DriveGear v1 (Autodesk Fusion 360 design; units mm, degrees)
Autodesk Fusion 360 part; units mm, degrees
note: some values were not read from the file. Set by a fixed rule: which sketch regions a step uses.
sketch "Sketch1" plane through (0, 0, 0) normal (0, 1, 0) x (1, 0, 0)
  line L0 (25.6646, 0) -> (28.2938, 0.0001)
  line L1 (28.2938, 0.0001) -> (28.3201, 0.001)
  line L2 (28.3201, 0.001) -> (28.3702, 0.0041)
  line L3 (28.3702, 0.0041) -> (28.4441, 0.0108)
  line L4 (28.4441, 0.0108) -> (28.5416, 0.0225)
  line L5 (28.5416, 0.0225) -> (28.6623, 0.0406)
  line L6 (28.6623, 0.0406) -> (28.806, 0.0665)
  line L7 (28.806, 0.0665) -> (28.9724, 0.1014)
  line L8 (28.9724, 0.1014) -> (29.1609, 0.1467)
  line L9 (29.1609, 0.1467) -> (29.3711, 0.2038)
  line L10 (29.3711, 0.2038) -> (29.6025, 0.2738)
  line L11 (29.6025, 0.2738) -> (29.8544, 0.3582)
  line L12 (29.8544, 0.3582) -> (30.1263, 0.4581)
  line L13 (30.1263, 0.4581) -> (30.4173, 0.5748)
  line L14 (30.4173, 0.5748) -> (30.7268, 0.7094)
  line L15 (30.7268, 0.7094) -> (31.0539, 0.8632)
  line L16 (31.0539, 0.8632) -> (31.3978, 1.0372)
  line L17 (31.3978, 1.0372) -> (31.7575, 1.2325)
  line L18 (31.7575, 1.2325) -> (32.132, 1.4503)
  line L19 (32.132, 1.4503) -> (32.5204, 1.6915)
  line L20 (32.5204, 1.6915) -> (32.9216, 1.9571)
  line L21 (32.9216, 1.9571) -> (33.3344, 2.248)
  line L22 (33.3344, 2.248) -> (33.7578, 2.5652)
  line L23 (33.7578, 2.5652) -> (34.1905, 2.9094)
  line L24 (34.1905, 2.9094) -> (34.6313, 3.2816)
  line L25 (34.6313, 3.2816) -> (35.0789, 3.6823)
  line L26 (35.0789, 3.6823) -> (35.532, 4.1124)
  line L27 (35.532, 4.1124) -> (35.9893, 4.5725)
  line L28 (35.9893, 4.5725) -> (36.4494, 5.0631)
  line L29 (36.4494, 5.0631) -> (36.6248, 5.5415)
  line L30 (36.6248, 5.5415) -> (36.4585, 6.5468)
  line L31 (36.4585, 6.5468) -> (36.1385, 6.9433)
  line L32 (36.1385, 6.9433) -> (35.5449, 7.2596)
  line L33 (35.5449, 7.2596) -> (34.9638, 7.5479)
  line L34 (34.9638, 7.5479) -> (34.3963, 7.8092)
  line L35 (34.3963, 7.8092) -> (33.8435, 8.0445)
  line L36 (33.8435, 8.0445) -> (33.3063, 8.2548)
  line L37 (33.3063, 8.2548) -> (32.7858, 8.4414)
  line L38 (32.7858, 8.4414) -> (32.2829, 8.6054)
  line L39 (32.2829, 8.6054) -> (31.7983, 8.7479)
  line L40 (31.7983, 8.7479) -> (31.333, 8.8702)
  line L41 (31.333, 8.8702) -> (30.8876, 8.9734)
  line L42 (30.8876, 8.9734) -> (30.4629, 9.059)
  line L43 (30.4629, 9.059) -> (30.0595, 9.1282)
  line L44 (30.0595, 9.1282) -> (29.6779, 9.1822)
  line L45 (29.6779, 9.1822) -> (29.3187, 9.2224)
  line L46 (29.3187, 9.2224) -> (28.9824, 9.2502)
  line L47 (28.9824, 9.2502) -> (28.6692, 9.267)
  line L48 (28.6692, 9.267) -> (28.3797, 9.274)
  line L49 (28.3797, 9.274) -> (28.114, 9.2727)
  line L50 (28.114, 9.2727) -> (27.8724, 9.2646)
  line L51 (27.8724, 9.2646) -> (27.655, 9.2509)
  line L52 (27.655, 9.2509) -> (27.4619, 9.2331)
  line L53 (27.4619, 9.2331) -> (27.2932, 9.2126)
  line L54 (27.2932, 9.2126) -> (27.1488, 9.1908)
  line L55 (27.1488, 9.1908) -> (27.0287, 9.169)
  line L56 (27.0287, 9.169) -> (26.9327, 9.1488)
  line L57 (26.9327, 9.1488) -> (26.8606, 9.1314)
  line L58 (26.8606, 9.1314) -> (26.8121, 9.1182)
  line L59 (26.8121, 9.1182) -> (26.7868, 9.1106)
  line L60 (26.7868, 9.1106) -> (24.2977, 8.264)
  line L61 (24.2977, 8.264) -> (22.2262, 12.8323)
  line L62 (22.2262, 12.8323) -> (24.5031, 14.1469)
  line L63 (24.5031, 14.1469) -> (24.5254, 14.1609)
  line L64 (24.5254, 14.1609) -> (24.5673, 14.1887)
  line L65 (24.5673, 14.1887) -> (24.6279, 14.2314)
  line L66 (24.6279, 14.2314) -> (24.7064, 14.2903)
  line L67 (24.7064, 14.2903) -> (24.802, 14.3664)
  line L68 (24.802, 14.3664) -> (24.9135, 14.4606)
  line L69 (24.9135, 14.4606) -> (25.0401, 14.574)
  line L70 (25.0401, 14.574) -> (25.1807, 14.7075)
  line L71 (25.1807, 14.7075) -> (25.3342, 14.862)
  line L72 (25.3342, 14.862) -> (25.4996, 15.0384)
  line L73 (25.4996, 15.0384) -> (25.6756, 15.2374)
  line L74 (25.6756, 15.2374) -> (25.8611, 15.4598)
  line L75 (25.8611, 15.4598) -> (26.0548, 15.7064)
  line L76 (26.0548, 15.7064) -> (26.2555, 15.9778)
  line L77 (26.2555, 15.9778) -> (26.4619, 16.2745)
  line L78 (26.4619, 16.2745) -> (26.6727, 16.5971)
  line L79 (26.6727, 16.5971) -> (26.8865, 16.9461)
  line L80 (26.8865, 16.9461) -> (27.102, 17.322)
  line L81 (27.102, 17.322) -> (27.3178, 17.7251)
  line L82 (27.3178, 17.7251) -> (27.5324, 18.1557)
  line L83 (27.5324, 18.1557) -> (27.7444, 18.614)
  line L84 (27.7444, 18.614) -> (27.9525, 19.1004)
  line L85 (27.9525, 19.1004) -> (28.1551, 19.6149)
  line L86 (28.1551, 19.6149) -> (28.3508, 20.1576)
  line L87 (28.3508, 20.1576) -> (28.538, 20.7284)
  line L88 (28.538, 20.7284) -> (28.7154, 21.3275)
  line L89 (28.7154, 21.3275) -> (28.8814, 21.9545)
  line L90 (28.8814, 21.9545) -> (29.0346, 22.6095)
  line L91 (29.0346, 22.6095) -> (28.9472, 23.1115)
  line L92 (28.9472, 23.1115) -> (28.3006, 23.8989)
  line L93 (28.3006, 23.8989) -> (27.8252, 24.0823)
  line L94 (27.8252, 24.0823) -> (27.1529, 24.0594)
  line L95 (27.1529, 24.0594) -> (26.5056, 24.0186)
  line L96 (26.5056, 24.0186) -> (25.8835, 23.9611)
  line L97 (25.8835, 23.9611) -> (25.2871, 23.8884)
  line L98 (25.2871, 23.8884) -> (24.7167, 23.802)
  line L99 (24.7167, 23.802) -> (24.1726, 23.7034)
  line L100 (24.1726, 23.7034) -> (23.6551, 23.5939)
  line L101 (23.6551, 23.5939) -> (23.1642, 23.4751)
  line L102 (23.1642, 23.4751) -> (22.7001, 23.3483)
  line L103 (22.7001, 23.3483) -> (22.2628, 23.2151)
  line L104 (22.2628, 23.2151) -> (21.8521, 23.0768)
  line L105 (21.8521, 23.0768) -> (21.4682, 22.935)
  line L106 (21.4682, 22.935) -> (21.1107, 22.791)
  line L107 (21.1107, 22.791) -> (20.7796, 22.6462)
  line L108 (20.7796, 22.6462) -> (20.4743, 22.5021)
  line L109 (20.4743, 22.5021) -> (20.1948, 22.36)
  line L110 (20.1948, 22.36) -> (19.9405, 22.2214)
  line L111 (19.9405, 22.2214) -> (19.7111, 22.0874)
  line L112 (19.7111, 22.0874) -> (19.5059, 21.9595)
  line L113 (19.5059, 21.9595) -> (19.3245, 21.839)
  line L114 (19.3245, 21.839) -> (19.1662, 21.7271)
  line L115 (19.1662, 21.7271) -> (19.0303, 21.625)
  line L116 (19.0303, 21.625) -> (18.9162, 21.5339)
  line L117 (18.9162, 21.5339) -> (18.823, 21.455)
  line L118 (18.823, 21.455) -> (18.75, 21.3894)
  line L119 (18.75, 21.3894) -> (18.6963, 21.3383)
  line L120 (18.6963, 21.3383) -> (18.6608, 21.3026)
  line L121 (18.6608, 21.3026) -> (18.6428, 21.2834)
  line L122 (18.6428, 21.2834) -> (16.9104, 19.3057)
  line L123 (16.9104, 19.3057) -> (12.8323, 22.2262)
  line L124 (12.8323, 22.2262) -> (14.1468, 24.5031)
  line L125 (14.1468, 24.5031) -> (14.1592, 24.5264)
  line L126 (14.1592, 24.5264) -> (14.1816, 24.5714)
  line L127 (14.1816, 24.5714) -> (14.2127, 24.6388)
  line L128 (14.2127, 24.6388) -> (14.2513, 24.729)
  line L129 (14.2513, 24.729) -> (14.2959, 24.8426)
  line L130 (14.2959, 24.8426) -> (14.3454, 24.98)
  line L131 (14.3454, 24.98) -> (14.3984, 25.1415)
  line L132 (14.3984, 25.1415) -> (14.4534, 25.3274)
  line L133 (14.4534, 25.3274) -> (14.5091, 25.538)
  line L134 (14.5091, 25.538) -> (14.5641, 25.7734)
  line L135 (14.5641, 25.7734) -> (14.617, 26.0338)
  line L136 (14.617, 26.0338) -> (14.6664, 26.3192)
  line L137 (14.6664, 26.3192) -> (14.7109, 26.6295)
  line L138 (14.7109, 26.6295) -> (14.7491, 26.9649)
  line L139 (14.7491, 26.9649) -> (14.7794, 27.3251)
  line L140 (14.7794, 27.3251) -> (14.8007, 27.7098)
  line L141 (14.8007, 27.7098) -> (14.8113, 28.119)
  line L142 (14.8113, 28.119) -> (14.81, 28.5523)
  line L143 (14.81, 28.5523) -> (14.7953, 29.0092)
  line L144 (14.7953, 29.0092) -> (14.7659, 29.4895)
  line L145 (14.7659, 29.4895) -> (14.7204, 29.9925)
  line L146 (14.7204, 29.9925) -> (14.6574, 30.5177)
  line L147 (14.6574, 30.5177) -> (14.5756, 31.0645)
  line L148 (14.5756, 31.0645) -> (14.4737, 31.6323)
  line L149 (14.4737, 31.6323) -> (14.3504, 32.2204)
  line L150 (14.3504, 32.2204) -> (14.2045, 32.8278)
  line L151 (14.2045, 32.8278) -> (14.0348, 33.4539)
  line L152 (14.0348, 33.4539) -> (13.8399, 34.0977)
  line L153 (13.8399, 34.0977) -> (13.5133, 34.4888)
  line L154 (13.5133, 34.4888) -> (12.5596, 34.8474)
  line L155 (12.5596, 34.8474) -> (12.0562, 34.7684)
  line L156 (12.0562, 34.7684) -> (11.4854, 34.4126)
  line L157 (11.4854, 34.4126) -> (10.9452, 34.0535)
  line L158 (10.9452, 34.0535) -> (10.4352, 33.6927)
  line L159 (10.4352, 33.6927) -> (9.955, 33.3315)
  line L160 (9.955, 33.3315) -> (9.5043, 32.9715)
  line L161 (9.5043, 32.9715) -> (9.0824, 32.6141)
  line L162 (9.0824, 32.6141) -> (8.6889, 32.2605)
  line L163 (8.6889, 32.2605) -> (8.3233, 31.9121)
  line L164 (8.3233, 31.9121) -> (7.9847, 31.5703)
  line L165 (7.9847, 31.5703) -> (7.6726, 31.2362)
  line L166 (7.6726, 31.2362) -> (7.3861, 30.9112)
  line L167 (7.3861, 30.9112) -> (7.1245, 30.5964)
  line L168 (7.1245, 30.5964) -> (6.8869, 30.2929)
  line L169 (6.8869, 30.2929) -> (6.6725, 30.002)
  line L170 (6.6725, 30.002) -> (6.4803, 29.7246)
  line L171 (6.4803, 29.7246) -> (6.3092, 29.4618)
  line L172 (6.3092, 29.4618) -> (6.1583, 29.2146)
  line L173 (6.1583, 29.2146) -> (6.0265, 28.9838)
  line L174 (6.0265, 28.9838) -> (5.9128, 28.7705)
  line L175 (5.9128, 28.7705) -> (5.816, 28.5754)
  line L176 (5.816, 28.5754) -> (5.7348, 28.3993)
  line L177 (5.7348, 28.3993) -> (5.6683, 28.2429)
  line L178 (5.6683, 28.2429) -> (5.615, 28.107)
  line L179 (5.615, 28.107) -> (5.5737, 27.9921)
  line L180 (5.5737, 27.9921) -> (5.5433, 27.8988)
  line L181 (5.5433, 27.8988) -> (5.5223, 27.8276)
  line L182 (5.5223, 27.8276) -> (5.5095, 27.779)
  line L183 (5.5095, 27.779) -> (5.5035, 27.7534)
  line L184 (5.5035, 27.7534) -> (4.992, 25.1744)
  line L185 (4.992, 25.1744) -> (0, 25.6646)
  line L186 (0, 25.6646) -> (-0.0001, 28.2938)
  line L187 (-0.0001, 28.2938) -> (-0.001, 28.3201)
  line L188 (-0.001, 28.3201) -> (-0.0041, 28.3702)
  line L189 (-0.0041, 28.3702) -> (-0.0108, 28.4441)
  line L190 (-0.0108, 28.4441) -> (-0.0225, 28.5416)
  line L191 (-0.0225, 28.5416) -> (-0.0406, 28.6623)
  line L192 (-0.0406, 28.6623) -> (-0.0665, 28.806)
  line L193 (-0.0665, 28.806) -> (-0.1014, 28.9724)
  line L194 (-0.1014, 28.9724) -> (-0.1467, 29.1609)
  line L195 (-0.1467, 29.1609) -> (-0.2038, 29.3711)
  line L196 (-0.2038, 29.3711) -> (-0.2738, 29.6025)
  line L197 (-0.2738, 29.6025) -> (-0.3582, 29.8544)
  line L198 (-0.3582, 29.8544) -> (-0.4581, 30.1263)
  line L199 (-0.4581, 30.1263) -> (-0.5748, 30.4173)
  line L200 (-0.5748, 30.4173) -> (-0.7094, 30.7268)
  line L201 (-0.7094, 30.7268) -> (-0.8632, 31.0539)
  line L202 (-0.8632, 31.0539) -> (-1.0372, 31.3978)
  line L203 (-1.0372, 31.3978) -> (-1.2325, 31.7575)
  line L204 (-1.2325, 31.7575) -> (-1.4503, 32.132)
  line L205 (-1.4503, 32.132) -> (-1.6915, 32.5204)
  line L206 (-1.6915, 32.5204) -> (-1.9571, 32.9216)
  line L207 (-1.9571, 32.9216) -> (-2.248, 33.3344)
  line L208 (-2.248, 33.3344) -> (-2.5652, 33.7578)
  line L209 (-2.5652, 33.7578) -> (-2.9094, 34.1905)
  line L210 (-2.9094, 34.1905) -> (-3.2816, 34.6313)
  line L211 (-3.2816, 34.6313) -> (-3.6823, 35.0789)
  line L212 (-3.6823, 35.0789) -> (-4.1124, 35.532)
  line L213 (-4.1124, 35.532) -> (-4.5725, 35.9893)
  line L214 (-4.5725, 35.9893) -> (-5.0631, 36.4494)
  line L215 (-5.0631, 36.4494) -> (-5.5415, 36.6248)
  line L216 (-5.5415, 36.6248) -> (-6.5468, 36.4585)
  line L217 (-6.5468, 36.4585) -> (-6.9433, 36.1385)
  line L218 (-6.9433, 36.1385) -> (-7.2596, 35.5449)
  line L219 (-7.2596, 35.5449) -> (-7.5479, 34.9638)
  line L220 (-7.5479, 34.9638) -> (-7.8092, 34.3963)
  line L221 (-7.8092, 34.3963) -> (-8.0445, 33.8435)
  line L222 (-8.0445, 33.8435) -> (-8.2548, 33.3063)
  line L223 (-8.2548, 33.3063) -> (-8.4414, 32.7858)
  line L224 (-8.4414, 32.7858) -> (-8.6054, 32.2829)
  line L225 (-8.6054, 32.2829) -> (-8.7479, 31.7983)
  line L226 (-8.7479, 31.7983) -> (-8.8702, 31.333)
  line L227 (-8.8702, 31.333) -> (-8.9734, 30.8876)
  line L228 (-8.9734, 30.8876) -> (-9.059, 30.4629)
  line L229 (-9.059, 30.4629) -> (-9.1282, 30.0595)
  line L230 (-9.1282, 30.0595) -> (-9.1822, 29.6779)
  line L231 (-9.1822, 29.6779) -> (-9.2224, 29.3187)
  line L232 (-9.2224, 29.3187) -> (-9.2502, 28.9824)
  line L233 (-9.2502, 28.9824) -> (-9.267, 28.6692)
  line L234 (-9.267, 28.6692) -> (-9.274, 28.3797)
  line L235 (-9.274, 28.3797) -> (-9.2727, 28.114)
  line L236 (-9.2727, 28.114) -> (-9.2646, 27.8724)
  line L237 (-9.2646, 27.8724) -> (-9.2509, 27.655)
  line L238 (-9.2509, 27.655) -> (-9.2331, 27.4619)
  line L239 (-9.2331, 27.4619) -> (-9.2126, 27.2932)
  line L240 (-9.2126, 27.2932) -> (-9.1908, 27.1488)
  line L241 (-9.1908, 27.1488) -> (-9.169, 27.0287)
  line L242 (-9.169, 27.0287) -> (-9.1488, 26.9327)
  line L243 (-9.1488, 26.9327) -> (-9.1314, 26.8606)
  line L244 (-9.1314, 26.8606) -> (-9.1182, 26.8121)
  line L245 (-9.1182, 26.8121) -> (-9.1106, 26.7868)
  line L246 (-9.1106, 26.7868) -> (-8.264, 24.2977)
  line L247 (-8.264, 24.2977) -> (-12.8323, 22.2262)
  line L248 (-12.8323, 22.2262) -> (-14.1469, 24.5031)
  line L249 (-14.1469, 24.5031) -> (-14.1609, 24.5254)
  line L250 (-14.1609, 24.5254) -> (-14.1887, 24.5673)
  line L251 (-14.1887, 24.5673) -> (-14.2314, 24.6279)
  line L252 (-14.2314, 24.6279) -> (-14.2903, 24.7064)
  line L253 (-14.2903, 24.7064) -> (-14.3664, 24.802)
  line L254 (-14.3664, 24.802) -> (-14.4606, 24.9135)
  line L255 (-14.4606, 24.9135) -> (-14.574, 25.0401)
  line L256 (-14.574, 25.0401) -> (-14.7075, 25.1807)
  line L257 (-14.7075, 25.1807) -> (-14.862, 25.3342)
  line L258 (-14.862, 25.3342) -> (-15.0384, 25.4996)
  line L259 (-15.0384, 25.4996) -> (-15.2374, 25.6756)
  line L260 (-15.2374, 25.6756) -> (-15.4598, 25.8611)
  line L261 (-15.4598, 25.8611) -> (-15.7064, 26.0548)
  line L262 (-15.7064, 26.0548) -> (-15.9778, 26.2555)
  line L263 (-15.9778, 26.2555) -> (-16.2745, 26.4619)
  line L264 (-16.2745, 26.4619) -> (-16.5971, 26.6727)
  line L265 (-16.5971, 26.6727) -> (-16.9461, 26.8865)
  line L266 (-16.9461, 26.8865) -> (-17.322, 27.102)
  line L267 (-17.322, 27.102) -> (-17.7251, 27.3178)
  line L268 (-17.7251, 27.3178) -> (-18.1557, 27.5324)
  line L269 (-18.1557, 27.5324) -> (-18.614, 27.7444)
  line L270 (-18.614, 27.7444) -> (-19.1004, 27.9525)
  line L271 (-19.1004, 27.9525) -> (-19.6149, 28.1551)
  line L272 (-19.6149, 28.1551) -> (-20.1576, 28.3508)
  line L273 (-20.1576, 28.3508) -> (-20.7284, 28.538)
  line L274 (-20.7284, 28.538) -> (-21.3275, 28.7154)
  line L275 (-21.3275, 28.7154) -> (-21.9545, 28.8814)
  line L276 (-21.9545, 28.8814) -> (-22.6095, 29.0346)
  line L277 (-22.6095, 29.0346) -> (-23.1115, 28.9472)
  line L278 (-23.1115, 28.9472) -> (-23.8989, 28.3006)
  line L279 (-23.8989, 28.3006) -> (-24.0823, 27.8252)
  line L280 (-24.0823, 27.8252) -> (-24.0594, 27.1529)
  line L281 (-24.0594, 27.1529) -> (-24.0186, 26.5056)
  line L282 (-24.0186, 26.5056) -> (-23.9611, 25.8835)
  line L283 (-23.9611, 25.8835) -> (-23.8884, 25.2871)
  line L284 (-23.8884, 25.2871) -> (-23.802, 24.7167)
  line L285 (-23.802, 24.7167) -> (-23.7034, 24.1726)
  line L286 (-23.7034, 24.1726) -> (-23.5939, 23.6551)
  line L287 (-23.5939, 23.6551) -> (-23.4751, 23.1642)
  line L288 (-23.4751, 23.1642) -> (-23.3483, 22.7001)
  line L289 (-23.3483, 22.7001) -> (-23.2151, 22.2628)
  line L290 (-23.2151, 22.2628) -> (-23.0768, 21.8521)
  line L291 (-23.0768, 21.8521) -> (-22.935, 21.4682)
  line L292 (-22.935, 21.4682) -> (-22.791, 21.1107)
  line L293 (-22.791, 21.1107) -> (-22.6462, 20.7796)
  line L294 (-22.6462, 20.7796) -> (-22.5021, 20.4743)
  line L295 (-22.5021, 20.4743) -> (-22.36, 20.1948)
  line L296 (-22.36, 20.1948) -> (-22.2214, 19.9405)
  line L297 (-22.2214, 19.9405) -> (-22.0874, 19.7111)
  line L298 (-22.0874, 19.7111) -> (-21.9595, 19.5059)
  line L299 (-21.9595, 19.5059) -> (-21.839, 19.3245)
  line L300 (-21.839, 19.3245) -> (-21.7271, 19.1662)
  line L301 (-21.7271, 19.1662) -> (-21.625, 19.0303)
  line L302 (-21.625, 19.0303) -> (-21.5339, 18.9162)
  line L303 (-21.5339, 18.9162) -> (-21.455, 18.823)
  line L304 (-21.455, 18.823) -> (-21.3894, 18.75)
  line L305 (-21.3894, 18.75) -> (-21.3383, 18.6963)
  line L306 (-21.3383, 18.6963) -> (-21.3026, 18.6608)
  line L307 (-21.3026, 18.6608) -> (-21.2834, 18.6428)
  line L308 (-21.2834, 18.6428) -> (-19.3057, 16.9104)
  line L309 (-19.3057, 16.9104) -> (-22.2262, 12.8323)
  line L310 (-22.2262, 12.8323) -> (-24.5031, 14.1468)
  line L311 (-24.5031, 14.1468) -> (-24.5264, 14.1592)
  line L312 (-24.5264, 14.1592) -> (-24.5714, 14.1816)
  line L313 (-24.5714, 14.1816) -> (-24.6388, 14.2127)
  line L314 (-24.6388, 14.2127) -> (-24.729, 14.2513)
  line L315 (-24.729, 14.2513) -> (-24.8426, 14.2959)
  line L316 (-24.8426, 14.2959) -> (-24.98, 14.3454)
  line L317 (-24.98, 14.3454) -> (-25.1415, 14.3984)
  line L318 (-25.1415, 14.3984) -> (-25.3274, 14.4534)
  line L319 (-25.3274, 14.4534) -> (-25.538, 14.5091)
  line L320 (-25.538, 14.5091) -> (-25.7734, 14.5641)
  line L321 (-25.7734, 14.5641) -> (-26.0338, 14.617)
  line L322 (-26.0338, 14.617) -> (-26.3192, 14.6664)
  line L323 (-26.3192, 14.6664) -> (-26.6295, 14.7109)
  line L324 (-26.6295, 14.7109) -> (-26.9649, 14.7491)
  line L325 (-26.9649, 14.7491) -> (-27.3251, 14.7794)
  line L326 (-27.3251, 14.7794) -> (-27.7098, 14.8007)
  line L327 (-27.7098, 14.8007) -> (-28.119, 14.8113)
  line L328 (-28.119, 14.8113) -> (-28.5523, 14.81)
  line L329 (-28.5523, 14.81) -> (-29.0092, 14.7953)
  line L330 (-29.0092, 14.7953) -> (-29.4895, 14.7659)
  line L331 (-29.4895, 14.7659) -> (-29.9925, 14.7204)
  line L332 (-29.9925, 14.7204) -> (-30.5177, 14.6574)
  line L333 (-30.5177, 14.6574) -> (-31.0645, 14.5756)
  line L334 (-31.0645, 14.5756) -> (-31.6323, 14.4737)
  line L335 (-31.6323, 14.4737) -> (-32.2204, 14.3504)
  line L336 (-32.2204, 14.3504) -> (-32.8278, 14.2045)
  line L337 (-32.8278, 14.2045) -> (-33.4539, 14.0348)
  line L338 (-33.4539, 14.0348) -> (-34.0977, 13.8399)
  line L339 (-34.0977, 13.8399) -> (-34.4888, 13.5133)
  line L340 (-34.4888, 13.5133) -> (-34.8474, 12.5596)
  line L341 (-34.8474, 12.5596) -> (-34.7684, 12.0562)
  line L342 (-34.7684, 12.0562) -> (-34.4126, 11.4854)
  line L343 (-34.4126, 11.4854) -> (-34.0535, 10.9452)
  line L344 (-34.0535, 10.9452) -> (-33.6927, 10.4352)
  line L345 (-33.6927, 10.4352) -> (-33.3315, 9.955)
  line L346 (-33.3315, 9.955) -> (-32.9715, 9.5043)
  line L347 (-32.9715, 9.5043) -> (-32.6141, 9.0824)
  line L348 (-32.6141, 9.0824) -> (-32.2605, 8.6889)
  line L349 (-32.2605, 8.6889) -> (-31.9121, 8.3233)
  line L350 (-31.9121, 8.3233) -> (-31.5703, 7.9847)
  line L351 (-31.5703, 7.9847) -> (-31.2362, 7.6726)
  line L352 (-31.2362, 7.6726) -> (-30.9112, 7.3861)
  line L353 (-30.9112, 7.3861) -> (-30.5964, 7.1245)
  line L354 (-30.5964, 7.1245) -> (-30.2929, 6.8869)
  line L355 (-30.2929, 6.8869) -> (-30.002, 6.6725)
  line L356 (-30.002, 6.6725) -> (-29.7246, 6.4803)
  line L357 (-29.7246, 6.4803) -> (-29.4618, 6.3092)
  line L358 (-29.4618, 6.3092) -> (-29.2146, 6.1583)
  line L359 (-29.2146, 6.1583) -> (-28.9838, 6.0265)
  line L360 (-28.9838, 6.0265) -> (-28.7705, 5.9128)
  line L361 (-28.7705, 5.9128) -> (-28.5754, 5.816)
  line L362 (-28.5754, 5.816) -> (-28.3993, 5.7348)
  line L363 (-28.3993, 5.7348) -> (-28.2429, 5.6683)
  line L364 (-28.2429, 5.6683) -> (-28.107, 5.615)
  line L365 (-28.107, 5.615) -> (-27.9921, 5.5737)
  line L366 (-27.9921, 5.5737) -> (-27.8988, 5.5433)
  line L367 (-27.8988, 5.5433) -> (-27.8276, 5.5223)
  line L368 (-27.8276, 5.5223) -> (-27.779, 5.5095)
  line L369 (-27.779, 5.5095) -> (-27.7534, 5.5035)
  line L370 (-27.7534, 5.5035) -> (-25.1744, 4.992)
  line L371 (-25.1744, 4.992) -> (-25.6646, 0)
  line L372 (-25.6646, 0) -> (-28.2938, -0.0001)
  line L373 (-28.2938, -0.0001) -> (-28.3201, -0.001)
  line L374 (-28.3201, -0.001) -> (-28.3702, -0.0041)
  line L375 (-28.3702, -0.0041) -> (-28.4441, -0.0108)
  line L376 (-28.4441, -0.0108) -> (-28.5416, -0.0225)
  line L377 (-28.5416, -0.0225) -> (-28.6623, -0.0406)
  line L378 (-28.6623, -0.0406) -> (-28.806, -0.0665)
  line L379 (-28.806, -0.0665) -> (-28.9724, -0.1014)
  line L380 (-28.9724, -0.1014) -> (-29.1609, -0.1467)
  line L381 (-29.1609, -0.1467) -> (-29.3711, -0.2038)
  line L382 (-29.3711, -0.2038) -> (-29.6025, -0.2738)
  line L383 (-29.6025, -0.2738) -> (-29.8544, -0.3582)
  line L384 (-29.8544, -0.3582) -> (-30.1263, -0.4581)
  line L385 (-30.1263, -0.4581) -> (-30.4173, -0.5748)
  line L386 (-30.4173, -0.5748) -> (-30.7268, -0.7094)
  line L387 (-30.7268, -0.7094) -> (-31.0539, -0.8632)
  line L388 (-31.0539, -0.8632) -> (-31.3978, -1.0372)
  line L389 (-31.3978, -1.0372) -> (-31.7575, -1.2325)
  line L390 (-31.7575, -1.2325) -> (-32.132, -1.4503)
  line L391 (-32.132, -1.4503) -> (-32.5204, -1.6915)
  line L392 (-32.5204, -1.6915) -> (-32.9216, -1.9571)
  line L393 (-32.9216, -1.9571) -> (-33.3344, -2.248)
  line L394 (-33.3344, -2.248) -> (-33.7578, -2.5652)
  line L395 (-33.7578, -2.5652) -> (-34.1905, -2.9094)
  line L396 (-34.1905, -2.9094) -> (-34.6313, -3.2816)
  line L397 (-34.6313, -3.2816) -> (-35.0789, -3.6823)
  line L398 (-35.0789, -3.6823) -> (-35.532, -4.1124)
  line L399 (-35.532, -4.1124) -> (-35.9893, -4.5725)
  line L400 (-35.9893, -4.5725) -> (-36.4494, -5.0631)
  line L401 (-36.4494, -5.0631) -> (-36.6248, -5.5415)
  line L402 (-36.6248, -5.5415) -> (-36.4585, -6.5468)
  line L403 (-36.4585, -6.5468) -> (-36.1385, -6.9433)
  line L404 (-36.1385, -6.9433) -> (-35.5449, -7.2596)
  line L405 (-35.5449, -7.2596) -> (-34.9638, -7.5479)
  line L406 (-34.9638, -7.5479) -> (-34.3963, -7.8092)
  line L407 (-34.3963, -7.8092) -> (-33.8435, -8.0445)
  line L408 (-33.8435, -8.0445) -> (-33.3063, -8.2548)
  line L409 (-33.3063, -8.2548) -> (-32.7858, -8.4414)
  line L410 (-32.7858, -8.4414) -> (-32.2829, -8.6054)
  line L411 (-32.2829, -8.6054) -> (-31.7983, -8.7479)
  line L412 (-31.7983, -8.7479) -> (-31.333, -8.8702)
  line L413 (-31.333, -8.8702) -> (-30.8876, -8.9734)
  line L414 (-30.8876, -8.9734) -> (-30.4629, -9.059)
  line L415 (-30.4629, -9.059) -> (-30.0595, -9.1282)
  line L416 (-30.0595, -9.1282) -> (-29.6779, -9.1822)
  line L417 (-29.6779, -9.1822) -> (-29.3187, -9.2224)
  line L418 (-29.3187, -9.2224) -> (-28.9824, -9.2502)
  line L419 (-28.9824, -9.2502) -> (-28.6692, -9.267)
  line L420 (-28.6692, -9.267) -> (-28.3797, -9.274)
  line L421 (-28.3797, -9.274) -> (-28.114, -9.2727)
  line L422 (-28.114, -9.2727) -> (-27.8724, -9.2646)
  line L423 (-27.8724, -9.2646) -> (-27.655, -9.2509)
  line L424 (-27.655, -9.2509) -> (-27.4619, -9.2331)
  line L425 (-27.4619, -9.2331) -> (-27.2932, -9.2126)
  line L426 (-27.2932, -9.2126) -> (-27.1488, -9.1908)
  line L427 (-27.1488, -9.1908) -> (-27.0287, -9.169)
  line L428 (-27.0287, -9.169) -> (-26.9327, -9.1488)
  line L429 (-26.9327, -9.1488) -> (-26.8606, -9.1314)
  line L430 (-26.8606, -9.1314) -> (-26.8121, -9.1182)
  line L431 (-26.8121, -9.1182) -> (-26.7868, -9.1106)
  line L432 (-26.7868, -9.1106) -> (-24.2977, -8.264)
  line L433 (-24.2977, -8.264) -> (-22.2262, -12.8323)
  line L434 (-22.2262, -12.8323) -> (-24.5031, -14.1469)
  line L435 (-24.5031, -14.1469) -> (-24.5254, -14.1609)
  line L436 (-24.5254, -14.1609) -> (-24.5673, -14.1887)
  line L437 (-24.5673, -14.1887) -> (-24.6279, -14.2314)
  line L438 (-24.6279, -14.2314) -> (-24.7064, -14.2903)
  line L439 (-24.7064, -14.2903) -> (-24.802, -14.3664)
  line L440 (-24.802, -14.3664) -> (-24.9135, -14.4606)
  line L441 (-24.9135, -14.4606) -> (-25.0401, -14.574)
  line L442 (-25.0401, -14.574) -> (-25.1807, -14.7075)
  line L443 (-25.1807, -14.7075) -> (-25.3342, -14.862)
  line L444 (-25.3342, -14.862) -> (-25.4996, -15.0384)
  line L445 (-25.4996, -15.0384) -> (-25.6756, -15.2374)
  line L446 (-25.6756, -15.2374) -> (-25.8611, -15.4598)
  line L447 (-25.8611, -15.4598) -> (-26.0548, -15.7064)
  line L448 (-26.0548, -15.7064) -> (-26.2555, -15.9778)
  line L449 (-26.2555, -15.9778) -> (-26.4619, -16.2745)
  line L450 (-26.4619, -16.2745) -> (-26.6727, -16.5971)
  line L451 (-26.6727, -16.5971) -> (-26.8865, -16.9461)
  line L452 (-26.8865, -16.9461) -> (-27.102, -17.322)
  line L453 (-27.102, -17.322) -> (-27.3178, -17.7251)
  line L454 (-27.3178, -17.7251) -> (-27.5324, -18.1557)
  line L455 (-27.5324, -18.1557) -> (-27.7444, -18.614)
  line L456 (-27.7444, -18.614) -> (-27.9525, -19.1004)
  line L457 (-27.9525, -19.1004) -> (-28.1551, -19.6149)
  line L458 (-28.1551, -19.6149) -> (-28.3508, -20.1576)
  line L459 (-28.3508, -20.1576) -> (-28.538, -20.7284)
  line L460 (-28.538, -20.7284) -> (-28.7154, -21.3275)
  line L461 (-28.7154, -21.3275) -> (-28.8814, -21.9545)
  line L462 (-28.8814, -21.9545) -> (-29.0346, -22.6095)
  line L463 (-29.0346, -22.6095) -> (-28.9472, -23.1115)
  line L464 (-28.9472, -23.1115) -> (-28.3006, -23.8989)
  line L465 (-28.3006, -23.8989) -> (-27.8252, -24.0823)
  line L466 (-27.8252, -24.0823) -> (-27.1529, -24.0594)
  line L467 (-27.1529, -24.0594) -> (-26.5056, -24.0186)
  line L468 (-26.5056, -24.0186) -> (-25.8835, -23.9611)
  line L469 (-25.8835, -23.9611) -> (-25.2871, -23.8884)
  line L470 (-25.2871, -23.8884) -> (-24.7167, -23.802)
  line L471 (-24.7167, -23.802) -> (-24.1726, -23.7034)
  line L472 (-24.1726, -23.7034) -> (-23.6551, -23.5939)
  line L473 (-23.6551, -23.5939) -> (-23.1642, -23.4751)
  line L474 (-23.1642, -23.4751) -> (-22.7001, -23.3483)
  line L475 (-22.7001, -23.3483) -> (-22.2628, -23.2151)
  line L476 (-22.2628, -23.2151) -> (-21.8521, -23.0768)
  line L477 (-21.8521, -23.0768) -> (-21.4682, -22.935)
  line L478 (-21.4682, -22.935) -> (-21.1107, -22.791)
  line L479 (-21.1107, -22.791) -> (-20.7796, -22.6462)
  line L480 (-20.7796, -22.6462) -> (-20.4743, -22.5021)
  line L481 (-20.4743, -22.5021) -> (-20.1948, -22.36)
  line L482 (-20.1948, -22.36) -> (-19.9405, -22.2214)
  line L483 (-19.9405, -22.2214) -> (-19.7111, -22.0874)
  line L484 (-19.7111, -22.0874) -> (-19.5059, -21.9595)
  line L485 (-19.5059, -21.9595) -> (-19.3245, -21.839)
  line L486 (-19.3245, -21.839) -> (-19.1662, -21.7271)
  line L487 (-19.1662, -21.7271) -> (-19.0303, -21.625)
  line L488 (-19.0303, -21.625) -> (-18.9162, -21.5339)
  line L489 (-18.9162, -21.5339) -> (-18.823, -21.455)
  line L490 (-18.823, -21.455) -> (-18.75, -21.3894)
  line L491 (-18.75, -21.3894) -> (-18.6963, -21.3383)
  line L492 (-18.6963, -21.3383) -> (-18.6608, -21.3026)
  line L493 (-18.6608, -21.3026) -> (-18.6428, -21.2834)
  line L494 (-18.6428, -21.2834) -> (-16.9104, -19.3057)
  line L495 (-16.9104, -19.3057) -> (-12.8323, -22.2262)
  line L496 (-12.8323, -22.2262) -> (-14.1468, -24.5031)
  line L497 (-14.1468, -24.5031) -> (-14.1592, -24.5264)
  line L498 (-14.1592, -24.5264) -> (-14.1816, -24.5714)
  line L499 (-14.1816, -24.5714) -> (-14.2127, -24.6388)
  line L500 (-14.2127, -24.6388) -> (-14.2513, -24.729)
  line L501 (-14.2513, -24.729) -> (-14.2959, -24.8426)
  line L502 (-14.2959, -24.8426) -> (-14.3454, -24.98)
  line L503 (-14.3454, -24.98) -> (-14.3984, -25.1415)
  line L504 (-14.3984, -25.1415) -> (-14.4534, -25.3274)
  line L505 (-14.4534, -25.3274) -> (-14.5091, -25.538)
  line L506 (-14.5091, -25.538) -> (-14.5641, -25.7734)
  line L507 (-14.5641, -25.7734) -> (-14.617, -26.0338)
  line L508 (-14.617, -26.0338) -> (-14.6664, -26.3192)
  line L509 (-14.6664, -26.3192) -> (-14.7109, -26.6295)
  line L510 (-14.7109, -26.6295) -> (-14.7491, -26.9649)
  line L511 (-14.7491, -26.9649) -> (-14.7794, -27.3251)
  line L512 (-14.7794, -27.3251) -> (-14.8007, -27.7098)
  line L513 (-14.8007, -27.7098) -> (-14.8113, -28.119)
  line L514 (-14.8113, -28.119) -> (-14.81, -28.5523)
  line L515 (-14.81, -28.5523) -> (-14.7953, -29.0092)
  line L516 (-14.7953, -29.0092) -> (-14.7659, -29.4895)
  line L517 (-14.7659, -29.4895) -> (-14.7204, -29.9925)
  line L518 (-14.7204, -29.9925) -> (-14.6574, -30.5177)
  line L519 (-14.6574, -30.5177) -> (-14.5756, -31.0645)
  line L520 (-14.5756, -31.0645) -> (-14.4737, -31.6323)
  line L521 (-14.4737, -31.6323) -> (-14.3504, -32.2204)
  line L522 (-14.3504, -32.2204) -> (-14.2045, -32.8278)
  line L523 (-14.2045, -32.8278) -> (-14.0348, -33.4539)
  line L524 (-14.0348, -33.4539) -> (-13.8399, -34.0977)
  line L525 (-13.8399, -34.0977) -> (-13.5133, -34.4888)
  line L526 (-13.5133, -34.4888) -> (-12.5596, -34.8474)
  line L527 (-12.5596, -34.8474) -> (-12.0562, -34.7684)
  line L528 (-12.0562, -34.7684) -> (-11.4854, -34.4126)
  line L529 (-11.4854, -34.4126) -> (-10.9452, -34.0535)
  line L530 (-10.9452, -34.0535) -> (-10.4352, -33.6927)
  line L531 (-10.4352, -33.6927) -> (-9.955, -33.3315)
  line L532 (-9.955, -33.3315) -> (-9.5043, -32.9715)
  line L533 (-9.5043, -32.9715) -> (-9.0824, -32.6141)
  line L534 (-9.0824, -32.6141) -> (-8.6889, -32.2605)
  line L535 (-8.6889, -32.2605) -> (-8.3233, -31.9121)
  line L536 (-8.3233, -31.9121) -> (-7.9847, -31.5703)
  line L537 (-7.9847, -31.5703) -> (-7.6726, -31.2362)
  line L538 (-7.6726, -31.2362) -> (-7.3861, -30.9112)
  line L539 (-7.3861, -30.9112) -> (-7.1245, -30.5964)
  line L540 (-7.1245, -30.5964) -> (-6.8869, -30.2929)
  line L541 (-6.8869, -30.2929) -> (-6.6725, -30.002)
  line L542 (-6.6725, -30.002) -> (-6.4803, -29.7246)
  line L543 (-6.4803, -29.7246) -> (-6.3092, -29.4618)
  line L544 (-6.3092, -29.4618) -> (-6.1583, -29.2146)
  line L545 (-6.1583, -29.2146) -> (-6.0265, -28.9838)
  line L546 (-6.0265, -28.9838) -> (-5.9128, -28.7705)
  line L547 (-5.9128, -28.7705) -> (-5.816, -28.5754)
  line L548 (-5.816, -28.5754) -> (-5.7348, -28.3993)
  line L549 (-5.7348, -28.3993) -> (-5.6683, -28.2429)
  line L550 (-5.6683, -28.2429) -> (-5.615, -28.107)
  line L551 (-5.615, -28.107) -> (-5.5737, -27.9921)
  line L552 (-5.5737, -27.9921) -> (-5.5433, -27.8988)
  line L553 (-5.5433, -27.8988) -> (-5.5223, -27.8276)
  line L554 (-5.5223, -27.8276) -> (-5.5095, -27.779)
  line L555 (-5.5095, -27.779) -> (-5.5035, -27.7534)
  line L556 (-5.5035, -27.7534) -> (-4.992, -25.1744)
  line L557 (-4.992, -25.1744) -> (0, -25.6646)
  line L558 (0, -25.6646) -> (0.0001, -28.2938)
  line L559 (0.0001, -28.2938) -> (0.001, -28.3201)
  line L560 (0.001, -28.3201) -> (0.0041, -28.3702)
  line L561 (0.0041, -28.3702) -> (0.0108, -28.4441)
  line L562 (0.0108, -28.4441) -> (0.0225, -28.5416)
  line L563 (0.0225, -28.5416) -> (0.0406, -28.6623)
  line L564 (0.0406, -28.6623) -> (0.0665, -28.806)
  line L565 (0.0665, -28.806) -> (0.1014, -28.9724)
  line L566 (0.1014, -28.9724) -> (0.1467, -29.1609)
  line L567 (0.1467, -29.1609) -> (0.2038, -29.3711)
  line L568 (0.2038, -29.3711) -> (0.2738, -29.6025)
  line L569 (0.2738, -29.6025) -> (0.3582, -29.8544)
  line L570 (0.3582, -29.8544) -> (0.4581, -30.1263)
  line L571 (0.4581, -30.1263) -> (0.5748, -30.4173)
  line L572 (0.5748, -30.4173) -> (0.7094, -30.7268)
  line L573 (0.7094, -30.7268) -> (0.8632, -31.0539)
  line L574 (0.8632, -31.0539) -> (1.0372, -31.3978)
  line L575 (1.0372, -31.3978) -> (1.2325, -31.7575)
  line L576 (1.2325, -31.7575) -> (1.4503, -32.132)
  line L577 (1.4503, -32.132) -> (1.6915, -32.5204)
  line L578 (1.6915, -32.5204) -> (1.9571, -32.9216)
  line L579 (1.9571, -32.9216) -> (2.248, -33.3344)
  line L580 (2.248, -33.3344) -> (2.5652, -33.7578)
  line L581 (2.5652, -33.7578) -> (2.9094, -34.1905)
  line L582 (2.9094, -34.1905) -> (3.2816, -34.6313)
  line L583 (3.2816, -34.6313) -> (3.6823, -35.0789)
  line L584 (3.6823, -35.0789) -> (4.1124, -35.532)
  line L585 (4.1124, -35.532) -> (4.5725, -35.9893)
  line L586 (4.5725, -35.9893) -> (5.0631, -36.4494)
  line L587 (5.0631, -36.4494) -> (5.5415, -36.6248)
  line L588 (5.5415, -36.6248) -> (6.5468, -36.4585)
  line L589 (6.5468, -36.4585) -> (6.9433, -36.1385)
  line L590 (6.9433, -36.1385) -> (7.2596, -35.5449)
  line L591 (7.2596, -35.5449) -> (7.5479, -34.9638)
  line L592 (7.5479, -34.9638) -> (7.8092, -34.3963)
  line L593 (7.8092, -34.3963) -> (8.0445, -33.8435)
  line L594 (8.0445, -33.8435) -> (8.2548, -33.3063)
  line L595 (8.2548, -33.3063) -> (8.4414, -32.7858)
  line L596 (8.4414, -32.7858) -> (8.6054, -32.2829)
  line L597 (8.6054, -32.2829) -> (8.7479, -31.7983)
  line L598 (8.7479, -31.7983) -> (8.8702, -31.333)
  line L599 (8.8702, -31.333) -> (8.9734, -30.8876)
  line L600 (8.9734, -30.8876) -> (9.059, -30.4629)
  line L601 (9.059, -30.4629) -> (9.1282, -30.0595)
  line L602 (9.1282, -30.0595) -> (9.1822, -29.6779)
  line L603 (9.1822, -29.6779) -> (9.2224, -29.3187)
  line L604 (9.2224, -29.3187) -> (9.2502, -28.9824)
  line L605 (9.2502, -28.9824) -> (9.267, -28.6692)
  line L606 (9.267, -28.6692) -> (9.274, -28.3797)
  line L607 (9.274, -28.3797) -> (9.2727, -28.114)
  line L608 (9.2727, -28.114) -> (9.2646, -27.8724)
  line L609 (9.2646, -27.8724) -> (9.2509, -27.655)
  line L610 (9.2509, -27.655) -> (9.2331, -27.4619)
  line L611 (9.2331, -27.4619) -> (9.2126, -27.2932)
  line L612 (9.2126, -27.2932) -> (9.1908, -27.1488)
  line L613 (9.1908, -27.1488) -> (9.169, -27.0287)
  line L614 (9.169, -27.0287) -> (9.1488, -26.9327)
  line L615 (9.1488, -26.9327) -> (9.1314, -26.8606)
  line L616 (9.1314, -26.8606) -> (9.1182, -26.8121)
  line L617 (9.1182, -26.8121) -> (9.1106, -26.7868)
  line L618 (9.1106, -26.7868) -> (8.264, -24.2977)
  line L619 (8.264, -24.2977) -> (12.8323, -22.2262)
  line L620 (12.8323, -22.2262) -> (14.1469, -24.5031)
  line L621 (14.1469, -24.5031) -> (14.1609, -24.5254)
  line L622 (14.1609, -24.5254) -> (14.1887, -24.5673)
  line L623 (14.1887, -24.5673) -> (14.2314, -24.6279)
  line L624 (14.2314, -24.6279) -> (14.2903, -24.7064)
  line L625 (14.2903, -24.7064) -> (14.3664, -24.802)
  line L626 (14.3664, -24.802) -> (14.4606, -24.9135)
  line L627 (14.4606, -24.9135) -> (14.574, -25.0401)
  line L628 (14.574, -25.0401) -> (14.7075, -25.1807)
  line L629 (14.7075, -25.1807) -> (14.862, -25.3342)
  line L630 (14.862, -25.3342) -> (15.0384, -25.4996)
  line L631 (15.0384, -25.4996) -> (15.2374, -25.6756)
  line L632 (15.2374, -25.6756) -> (15.4598, -25.8611)
  line L633 (15.4598, -25.8611) -> (15.7064, -26.0548)
  line L634 (15.7064, -26.0548) -> (15.9778, -26.2555)
  line L635 (15.9778, -26.2555) -> (16.2745, -26.4619)
  line L636 (16.2745, -26.4619) -> (16.5971, -26.6727)
  line L637 (16.5971, -26.6727) -> (16.9461, -26.8865)
  line L638 (16.9461, -26.8865) -> (17.322, -27.102)
  line L639 (17.322, -27.102) -> (17.7251, -27.3178)
  line L640 (17.7251, -27.3178) -> (18.1557, -27.5324)
  line L641 (18.1557, -27.5324) -> (18.614, -27.7444)
  line L642 (18.614, -27.7444) -> (19.1004, -27.9525)
  line L643 (19.1004, -27.9525) -> (19.6149, -28.1551)
  line L644 (19.6149, -28.1551) -> (20.1576, -28.3508)
  line L645 (20.1576, -28.3508) -> (20.7284, -28.538)
  line L646 (20.7284, -28.538) -> (21.3275, -28.7154)
  line L647 (21.3275, -28.7154) -> (21.9545, -28.8814)
  line L648 (21.9545, -28.8814) -> (22.6095, -29.0346)
  line L649 (22.6095, -29.0346) -> (23.1115, -28.9472)
  line L650 (23.1115, -28.9472) -> (23.8989, -28.3006)
  line L651 (23.8989, -28.3006) -> (24.0823, -27.8252)
  line L652 (24.0823, -27.8252) -> (24.0594, -27.1529)
  line L653 (24.0594, -27.1529) -> (24.0186, -26.5056)
  line L654 (24.0186, -26.5056) -> (23.9611, -25.8835)
  line L655 (23.9611, -25.8835) -> (23.8884, -25.2871)
  line L656 (23.8884, -25.2871) -> (23.802, -24.7167)
  line L657 (23.802, -24.7167) -> (23.7034, -24.1726)
  line L658 (23.7034, -24.1726) -> (23.5939, -23.6551)
  line L659 (23.5939, -23.6551) -> (23.4751, -23.1642)
  line L660 (23.4751, -23.1642) -> (23.3483, -22.7001)
  line L661 (23.3483, -22.7001) -> (23.2151, -22.2628)
  line L662 (23.2151, -22.2628) -> (23.0768, -21.8521)
  line L663 (23.0768, -21.8521) -> (22.935, -21.4682)
  line L664 (22.935, -21.4682) -> (22.791, -21.1107)
  line L665 (22.791, -21.1107) -> (22.6462, -20.7796)
  line L666 (22.6462, -20.7796) -> (22.5021, -20.4743)
  line L667 (22.5021, -20.4743) -> (22.36, -20.1948)
  line L668 (22.36, -20.1948) -> (22.2214, -19.9405)
  line L669 (22.2214, -19.9405) -> (22.0874, -19.7111)
  line L670 (22.0874, -19.7111) -> (21.9595, -19.5059)
  line L671 (21.9595, -19.5059) -> (21.839, -19.3245)
  line L672 (21.839, -19.3245) -> (21.7271, -19.1662)
  line L673 (21.7271, -19.1662) -> (21.625, -19.0303)
  line L674 (21.625, -19.0303) -> (21.5339, -18.9162)
  line L675 (21.5339, -18.9162) -> (21.455, -18.823)
  line L676 (21.455, -18.823) -> (21.3894, -18.75)
  line L677 (21.3894, -18.75) -> (21.3383, -18.6963)
  line L678 (21.3383, -18.6963) -> (21.3026, -18.6608)
  line L679 (21.3026, -18.6608) -> (21.2834, -18.6428)
  line L680 (21.2834, -18.6428) -> (19.3057, -16.9104)
  line L681 (19.3057, -16.9104) -> (22.2262, -12.8323)
  line L682 (22.2262, -12.8323) -> (24.5031, -14.1468)
  line L683 (24.5031, -14.1468) -> (24.5264, -14.1592)
  line L684 (24.5264, -14.1592) -> (24.5714, -14.1816)
  line L685 (24.5714, -14.1816) -> (24.6388, -14.2127)
  line L686 (24.6388, -14.2127) -> (24.729, -14.2513)
  line L687 (24.729, -14.2513) -> (24.8426, -14.2959)
  line L688 (24.8426, -14.2959) -> (24.98, -14.3454)
  line L689 (24.98, -14.3454) -> (25.1415, -14.3984)
  line L690 (25.1415, -14.3984) -> (25.3274, -14.4534)
  line L691 (25.3274, -14.4534) -> (25.538, -14.5091)
  line L692 (25.538, -14.5091) -> (25.7734, -14.5641)
  line L693 (25.7734, -14.5641) -> (26.0338, -14.617)
  line L694 (26.0338, -14.617) -> (26.3192, -14.6664)
  line L695 (26.3192, -14.6664) -> (26.6295, -14.7109)
  line L696 (26.6295, -14.7109) -> (26.9649, -14.7491)
  line L697 (26.9649, -14.7491) -> (27.3251, -14.7794)
  line L698 (27.3251, -14.7794) -> (27.7098, -14.8007)
  line L699 (27.7098, -14.8007) -> (28.119, -14.8113)
  line L700 (28.119, -14.8113) -> (28.5523, -14.81)
  line L701 (28.5523, -14.81) -> (29.0092, -14.7953)
  line L702 (29.0092, -14.7953) -> (29.4895, -14.7659)
  line L703 (29.4895, -14.7659) -> (29.9925, -14.7204)
  line L704 (29.9925, -14.7204) -> (30.5177, -14.6574)
  line L705 (30.5177, -14.6574) -> (31.0645, -14.5756)
  line L706 (31.0645, -14.5756) -> (31.6323, -14.4737)
  line L707 (31.6323, -14.4737) -> (32.2204, -14.3504)
  line L708 (32.2204, -14.3504) -> (32.8278, -14.2045)
  line L709 (32.8278, -14.2045) -> (33.4539, -14.0348)
  line L710 (33.4539, -14.0348) -> (34.0977, -13.8399)
  line L711 (34.0977, -13.8399) -> (34.4888, -13.5133)
  line L712 (34.4888, -13.5133) -> (34.8474, -12.5596)
  line L713 (34.8474, -12.5596) -> (34.7684, -12.0562)
  line L714 (34.7684, -12.0562) -> (34.4126, -11.4854)
  line L715 (34.4126, -11.4854) -> (34.0535, -10.9452)
  line L716 (34.0535, -10.9452) -> (33.6927, -10.4352)
  line L717 (33.6927, -10.4352) -> (33.3315, -9.955)
  line L718 (33.3315, -9.955) -> (32.9715, -9.5043)
  line L719 (32.9715, -9.5043) -> (32.6141, -9.0824)
  line L720 (32.6141, -9.0824) -> (32.2605, -8.6889)
  line L721 (32.2605, -8.6889) -> (31.9121, -8.3233)
  line L722 (31.9121, -8.3233) -> (31.5703, -7.9847)
  line L723 (31.5703, -7.9847) -> (31.2362, -7.6726)
  line L724 (31.2362, -7.6726) -> (30.9112, -7.3861)
  line L725 (30.9112, -7.3861) -> (30.5964, -7.1245)
  line L726 (30.5964, -7.1245) -> (30.2929, -6.8869)
  line L727 (30.2929, -6.8869) -> (30.002, -6.6725)
  line L728 (30.002, -6.6725) -> (29.7246, -6.4803)
  line L729 (29.7246, -6.4803) -> (29.4618, -6.3092)
  line L730 (29.4618, -6.3092) -> (29.2146, -6.1583)
  line L731 (29.2146, -6.1583) -> (28.9838, -6.0265)
  line L732 (28.9838, -6.0265) -> (28.7705, -5.9128)
  line L733 (28.7705, -5.9128) -> (28.5754, -5.816)
  line L734 (28.5754, -5.816) -> (28.3993, -5.7348)
  line L735 (28.3993, -5.7348) -> (28.2429, -5.6683)
  line L736 (28.2429, -5.6683) -> (28.107, -5.615)
  line L737 (28.107, -5.615) -> (27.9921, -5.5737)
  line L738 (27.9921, -5.5737) -> (27.8988, -5.5433)
  line L739 (27.8988, -5.5433) -> (27.8276, -5.5223)
  line L740 (27.8276, -5.5223) -> (27.779, -5.5095)
  line L741 (27.779, -5.5095) -> (27.7534, -5.5035)
  line L742 (27.7534, -5.5035) -> (25.1744, -4.992)
  line L743 (25.1744, -4.992) -> (25.6646, 0)
  line L744 (2.6458, 0) -> (-2.6458, 0)
  line L745 (0, -2.6458) -> (0, 2.6458)
  circle A0 centre (31.3244, 5.1812) radius 2.077
  circle A1 centre (0, 0) radius 31.75
  circle A2 centre (0, 0) radius 37.0417
  circle A3 centre (0, 0) radius 28.2893
  arc A4 (1.557, 1.4013) -> (0.6299, 1.9365) centre (0.1299, 0) ccw
  line L746 (1.9924, -1.6527) -> (1.557, -1.4013)
  arc A5 (2.057, -0.5352) -> (2.057, 0.5352) centre (0.1299, 0) ccw
  line L747 (0.6299, -2.4393) -> (0.6299, -1.9365)
  line L748 (-2.2325, 0.7866) -> (-1.7971, 0.5352)
  arc A6 (0.6299, -1.9365) -> (1.557, -1.4013) centre (0.1299, 0) ccw
  line L749 (-0.3701, 2.4393) -> (-0.3701, 1.9365)
  arc A7 (2.4924, 0.7866) -> (1.9924, 1.6527) centre (0.1299, 0) ccw
  line L750 (0.6299, 2.4393) -> (0.6299, 1.9365)
  line L751 (2.4924, 0.7866) -> (2.057, 0.5352)
  arc A8 (-1.7325, 1.6527) -> (-2.2325, 0.7866) centre (0.1299, 0) ccw
  line L752 (1.9924, 1.6527) -> (1.557, 1.4013)
  line L753 (2.4924, -0.7866) -> (2.057, -0.5352)
  line L754 (-0.3701, -2.4393) -> (-0.3701, -1.9365)
  line L755 (-1.7325, 1.6527) -> (-1.2971, 1.4013)
  arc A9 (-0.3701, -2.4393) -> (0.6299, -2.4393) centre (0.1299, 0) ccw
  arc A10 (1.9924, -1.6527) -> (2.4924, -0.7866) centre (0.1299, 0) ccw
  arc A11 (-0.3701, 1.9365) -> (-1.2971, 1.4013) centre (0.1299, 0) ccw
  arc A12 (-1.7971, 0.5352) -> (-1.7971, -0.5352) centre (0.1299, 0) ccw
  arc A13 (-1.2971, -1.4013) -> (-0.3701, -1.9365) centre (0.1299, 0) ccw
  line L756 (-2.2325, -0.7866) -> (-1.7971, -0.5352)
  arc A14 (-2.2325, -0.7866) -> (-1.7325, -1.6527) centre (0.1299, 0) ccw
  line L757 (-1.7325, -1.6527) -> (-1.2971, -1.4013)
  arc A15 (0.6299, 2.4393) -> (-0.3701, 2.4393) centre (0.1299, 0) ccw
extrude "Extrude1" add sketch "Sketch1" along normal blind 5 contours L0 L60 L61 L62 L122 L123 L124 L184 L185 L186 L246 L247 L248 L308 L309 L310 L370 L371 L372 L432 L433 L434 L494 L495 L496 L556 L557 L558 L618 L619 L620 L680 L681 L682 L742 L743 A3 | L0 L1 L2 L3 L4 L5 L6 L7 L8 L9 L10 L11 L12 L13 L14 L15 L16 L17 L43 L44 L45 L46 L47 L48 L49 L50 L51 L52 L53 L54 L55 L56 L57 L58 L59 L60 A0 A1 A3 | L682 L683 L684 L685 L686 L687 L688 L689 L690 L691 L692 L693 L694 L695 L696 L697 L698 L699 L725 L726 L727 L728 L729 L730 L731 L732 L733 L734 L735 L736 L737 L738 L739 L740 L741 L742 A1 A3 | L62 L63 L64 L65 L66 L67 L68 L69 L70 L71 L72 L73 L74 L75 L76 L77 L78 L79 L105 L106 L107 L108 L109 L110 L111 L112 L113 L114 L115 L116 L117 L118 L119 L120 L121 L122 A1 A3 | L620 L621 L622 L623 L624 L625 L626 L627 L628 L629 L630 L631 L632 L633 L634 L635 L636 L637 L663 L664 L665 L666 L667 L668 L669 L670 L671 L672 L673 L674 L675 L676 L677 L678 L679 L680 A1 A3 | L124 L125 L126 L127 L128 L129 L130 L131 L132 L133 L134 L135 L136 L137 L138 L139 L140 L141 L167 L168 L169 L170 L171 L172 L173 L174 L175 L176 L177 L178 L179 L180 L181 L182 L183 L184 A1 A3 | L558 L559 L560 L561 L562 L563 L564 L565 L566 L567 L568 L569 L570 L571 L572 L573 L574 L575 L601 L602 L603 L604 L605 L606 L607 L608 L609 L610 L611 L612 L613 L614 L615 L616 L617 L618 A1 A3 | L186 L187 L188 L189 L190 L191 L192 L193 L194 L195 L196 L197 L198 L199 L200 L201 L202 L203 L229 L230 L231 L232 L233 L234 L235 L236 L237 L238 L239 L240 L241 L242 L243 L244 L245 L246 A1 A3 | L496 L497 L498 L499 L500 L501 L502 L503 L504 L505 L506 L507 L508 L509 L510 L511 L512 L513 L539 L540 L541 L542 L543 L544 L545 L546 L547 L548 L549 L550 L551 L552 L553 L554 L555 L556 A1 A3 | L248 L249 L250 L251 L252 L253 L254 L255 L256 L257 L258 L259 L260 L261 L262 L263 L264 L265 L291 L292 L293 L294 L295 L296 L297 L298 L299 L300 L301 L302 L303 L304 L305 L306 L307 L308 A1 A3 | L434 L435 L436 L437 L438 L439 L440 L441 L442 L443 L444 L445 L446 L447 L448 L449 L450 L451 L477 L478 L479 L480 L481 L482 L483 L484 L485 L486 L487 L488 L489 L490 L491 L492 L493 L494 A1 A3 | L310 L311 L312 L313 L314 L315 L316 L317 L318 L319 L320 L321 L322 L323 L324 L325 L326 L327 L353 L354 L355 L356 L357 L358 L359 L360 L361 L362 L363 L364 L365 L366 L367 L368 L369 L370 A1 A3 | L372 L373 L374 L375 L376 L377 L378 L379 L380 L381 L382 L383 L384 L385 L386 L387 L388 L389 L415 L416 L417 L418 L419 L420 L421 L422 L423 L424 L425 L426 L427 L428 L429 L430 L431 L432 A1 A3 | L17 L18 L19 L20 L21 L22 L23 L24 L25 L26 L27 L28 L29 L30 L31 L32 L33 L34 L35 L36 L37 L38 L39 L40 L41 L42 L43 A0 A1 | A0 A1 | A0 A1 | L699 L700 L701 L702 L703 L704 L705 L706 L707 L708 L709 L710 L711 L712 L713 L714 L715 L716 L717 L718 L719 L720 L721 L722 L723 L724 L725 A1 | L79 L80 L81 L82 L83 L84 L85 L86 L87 L88 L89 L90 L91 L92 L93 L94 L95 L96 L97 L98 L99 L100 L101 L102 L103 L104 L105 A1 | L637 L638 L639 L640 L641 L642 L643 L644 L645 L646 L647 L648 L649 L650 L651 L652 L653 L654 L655 L656 L657 L658 L659 L660 L661 L662 L663 A1 | L141 L142 L143 L144 L145 L146 L147 L148 L149 L150 L151 L152 L153 L154 L155 L156 L157 L158 L159 L160 L161 L162 L163 L164 L165 L166 L167 A1 | L575 L576 L577 L578 L579 L580 L581 L582 L583 L584 L585 L586 L587 L588 L589 L590 L591 L592 L593 L594 L595 L596 L597 L598 L599 L600 L601 A1 | L203 L204 L205 L206 L207 L208 L209 L210 L211 L212 L213 L214 L215 L216 L217 L218 L219 L220 L221 L222 L223 L224 L225 L226 L227 L228 L229 A1 | L513 L514 L515 L516 L517 L518 L519 L520 L521 L522 L523 L524 L525 L526 L527 L528 L529 L530 L531 L532 L533 L534 L535 L536 L537 L538 L539 A1 | L265 L266 L267 L268 L269 L270 L271 L272 L273 L274 L275 L276 L277 L278 L279 L280 L281 L282 L283 L284 L285 L286 L287 L288 L289 L290 L291 A1 | L451 L452 L453 L454 L455 L456 L457 L458 L459 L460 L461 L462 L463 L464 L465 L466 L467 L468 L469 L470 L471 L472 L473 L474 L475 L476 L477 A1 | L327 L328 L329 L330 L331 L332 L333 L334 L335 L336 L337 L338 L339 L340 L341 L342 L343 L344 L345 L346 L347 L348 L349 L350 L351 L352 L353 A1 | L389 L390 L391 L392 L393 L394 L395 L396 L397 L398 L399 L400 L401 L402 L403 L404 L405 L406 L407 L408 L409 L410 L411 L412 L413 L414 L415 A1
